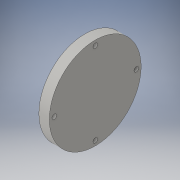
# Autodesk Inventor part: 100mm-FlangeBottom-Sketch
Saved by Autodesk Inventor 2016 SP1 (Build 200210100, 210)
## iProperties
Created: 2017-05-04
Part Number: 100mm-FlangeBottom-Sketch
Material: Generic
Document SubType Name: Modeling
Designer: ASUS
Density: 1 g/cm^3
Appearance: Default
Author: ASUS
Autodesk Inventor part; units mm, degrees
ref_plane "YZ Plane" through (0, 0, 0) normal (1, 0, 0) x (0, 1, 0)
ref_plane "XZ Plane" through (0, 0, 0) normal (0, 1, 0) x (-1, 0, 0)
ref_plane "XY Plane" through (0, 0, 0) normal (0, 0, 1) x (1, 0, 0)
sketch "Sketch4" plane through (0, 0, 0) normal (0, 1, 0) x (-1, 0, 0)
  line L0 (0, 0) -> (0, 66)
  line L1 (0, 66) -> (15, 66)
  line L2 (15, 66) -> (15, 50.5)
  line L3 (15, 50.5) -> (5, 50.5)
  line L4 (5, 50.5) -> (5, 46.5)
  line L5 (5, 46.5) -> (15, 46.5)
  line L6 (15, 46.5) -> (15, 0)
  line L7 (15, 0) -> (0, 0)
  dimension "d6" = 66
  dimension "d7" = 15
  dimension "d8" = 15.5
  dimension "d9" = 10
  dimension "d10" = 4
  constraints: 16 end point, 6 perpendicular, 2 vertical, 1 point on line
  measures "d6" distance of L0.start L0.end
  measures "d7" distance of L0.end L1.end
  measures "d8" distance of L1.end L2.end
  measures "d9" distance of L2.end L3.end
  measures "d10" distance of L3.end L4.end
revolve "Revolution1" add sketch "Sketch4" angle 360 about axis through (-15, 0, 0) along (1, 0, 0)
sketch "Sketch5" plane through (-15, 0, 0) normal (-1, 0, 0) x (0, 0, 1)
  point P0 (0, 0)
sketch "Sketch6" plane through (-15, 0, 0) normal (-1, 0, 0) x (0, 0, 1)
  circle A0 centre (0, 0) radius 59
  point P0 (59, 0)
  point P1 (0, -59)
  point P2 (-59, 0)
  point P3 (0, 59)
  dimension "d13" = 118
  constraints: 4 point on circle, 1 centre point, 1 coincident
  measures "d13" diameter of A0
hole "Hole1" at (-15, 0, 59) at (-15, -59, 0) at (-15, 0, -59) at (-15, 59, 0) direction (1, 0, 0) diameter 6.6 end through all clearance for "Flat Head Machine Screw" size "M6" standard "Ansi Metric M Profile"
body "Solid1"
